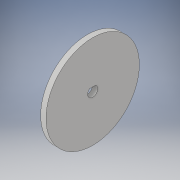
# Autodesk Inventor part: wheel_acry
Saved by Autodesk Inventor 2019 (Build 230136000, 136)
## iProperties
Created: 2018-09-07
Part Number: wheel_acry
Material: Generic
Document SubType Name: Modeling
Designer: mspet
Density: 1 g/cm^3
Appearance: Default
Author: mspet
Autodesk Inventor part; units mm, degrees
ref_plane "YZ Plane" through (0, 0, 0) normal (1, 0, 0) x (0, 1, 0)
ref_plane "XZ Plane" through (0, 0, 0) normal (0, 1, 0) x (-1, 0, 0)
ref_plane "XY Plane" through (0, 0, 0) normal (0, 0, 1) x (1, 0, 0)
sketch "Sketch1" plane through (0, 0, 0) normal (1, 0, 0) x (0, 1, 0)
  circle A0 centre (0, 0) radius 27.7622
  dimension "d0" = 55.5244
  constraints: 1 centre point, 1 coincident
  measures "d0" diameter of A0
extrude "Extrusion1" add sketch "Sketch1" along normal blind 3.175
sketch "Sketch2" plane through (3.175, 0, 0) normal (1, 0, 0) x (0, 0, -1)
  arc A0 (-1.8, 2.4) -> (1.8, 2.4) centre (0, 0) ccw
  line L0 (0, -3) -> (4.3918, -3) construction
  line L1 (-4.718, 2.4) -> (9.613, 2.4)
  dimension "d3" = 6
  dimension "d4" = 5.4
  constraints: 4 end point, 3 point on circle, 2 horizontal, 2 point on line, 1 centre point, 1 coincident
  measures "d3" diameter of A0
  measures "d4" distance between parallel lines of L0 L1
extrude "Extrusion2" cut sketch "Sketch2" against normal blind 3.175
body "Solid1"
